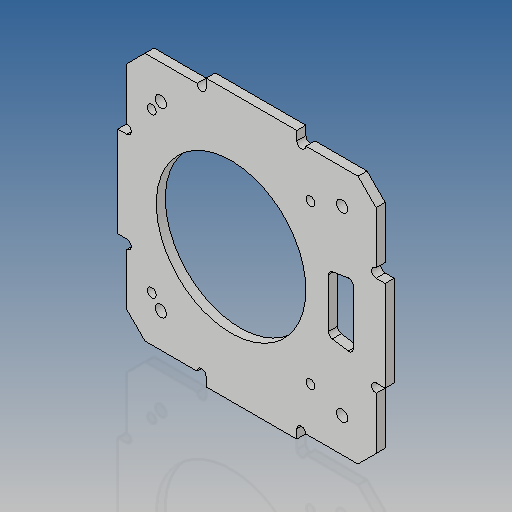
# Autodesk Inventor part: Pieza4
Saved by Autodesk Inventor 2017 (Build 210142000, 142)
## iProperties
Part Number: Pieza4
Material: Genérico
Document SubType Name: Modeling
Designer: Leo
Density: 1 g/cm^3
Appearance: Valor por defecto
Author: Leo
Autodesk Inventor part; units mm, degrees
ref_plane "YZ Plane" through (0, 0, 0) normal (1, 0, 0) x (0, 1, 0)
ref_plane "XZ Plane" through (0, 0, 0) normal (0, 1, 0) x (-1, 0, 0)
ref_plane "XY Plane" through (0, 0, 0) normal (0, 0, 1) x (1, 0, 0)
sketch "Boceto1" plane through (0, 0, 0) normal (0, 0, 1) x (1, 0, 0)
  line L0 (32.5, 7.5) -> (0.5, 7.5) construction
  line L1 (0.5, 7.5) -> (0.5, 31.5) construction
  line L2 (0.5, 31.5) -> (32.5, 31.5) construction
  line L3 (32.5, 31.5) -> (32.5, 7.5) construction
  line L4 (30, -12) -> (30, -31) construction
  line L5 (30, -31) -> (3, -31) construction
  line L6 (3, -31) -> (3, -12) construction
  line L7 (3, -12) -> (30, -12) construction
  circle A0 centre (-40, -40) radius 2.5 projected
  circle A1 centre (-40, 40) radius 2.5 projected
  circle A2 centre (40, 40) radius 2.5 projected
  circle A3 centre (40, -40) radius 2.5 projected
  line L8 (-59, 20) -> (-59, -20) projected
  line L9 (-59, -20) -> (-55, -20) projected
  arc A4 (-55, -24) -> (-55, -20) centre (-55, -22) ccw projected
  line L10 (-55, -24) -> (-55, -47) projected
  line L11 (-55, -47) -> (-47, -55) projected
  line L12 (-47, -55) -> (-24, -55) projected
  arc A5 (-20, -55) -> (-24, -55) centre (-22, -55) ccw projected
  line L13 (-20, -55) -> (-20, -59) projected
  line L14 (-20, -59) -> (20, -59) projected
  line L15 (20, -59) -> (20, -55) projected
  arc A6 (24, -55) -> (20, -55) centre (22, -55) ccw projected
  line L16 (24, -55) -> (47, -55) projected
  line L17 (47, -55) -> (55, -47) projected
  line L18 (55, -47) -> (55, -24) projected
  arc A7 (55, -20) -> (55, -24) centre (55, -22) ccw projected
  line L19 (55, -20) -> (59, -20) projected
  line L20 (59, -20) -> (59, 20) projected
  line L21 (59, 20) -> (55, 20) projected
  arc A8 (55, 24) -> (55, 20) centre (55, 22) ccw projected
  line L22 (55, 24) -> (55, 47) projected
  line L23 (55, 47) -> (47, 55) projected
  line L24 (47, 55) -> (24, 55) projected
  arc A9 (20, 55) -> (24, 55) centre (22, 55) ccw projected
  line L25 (20, 55) -> (20, 59) projected
  line L26 (20, 59) -> (-20, 59) projected
  line L27 (-20, 59) -> (-20, 55) projected
  arc A10 (-24, 55) -> (-20, 55) centre (-22, 55) ccw projected
  line L28 (-24, 55) -> (-47, 55) projected
  line L29 (-47, 55) -> (-55, 47) projected
  line L30 (-55, 47) -> (-55, 24) projected
  arc A11 (-55, 20) -> (-55, 24) centre (-55, 22) ccw projected
  line L31 (-55, 20) -> (-59, 20) projected
  line L32 (26, 35) -> (-44, 35) construction
  line L33 (-44, 35) -> (-44, -35) construction
  line L34 (-44, -35) -> (26, -35) construction
  line L35 (26, -35) -> (26, 35) construction
  circle A12 centre (26, 35) radius 2
  circle A13 centre (26, -35) radius 2
  circle A14 centre (-44, -35) radius 2
  circle A15 centre (-44, 35) radius 2
  circle A16 centre (-9, 0) radius 33
  line L36 (45, 12) -> (45, -12)
  arc A17 (42.6827, -13.9747) -> (45, -12) centre (43, -12) ccw
  line L37 (42.6827, -13.9747) -> (35.6827, -12.85)
  arc A18 (34, -10.8753) -> (35.6827, -12.85) centre (36, -10.8753) ccw
  line L38 (34, -10.8753) -> (34, 10.8753)
  arc A19 (35.6827, 12.85) -> (34, 10.8753) centre (36, 10.8753) ccw
  line L39 (35.6827, 12.85) -> (42.6827, 13.9747)
  arc A20 (45, 12) -> (42.6827, 13.9747) centre (43, 12) ccw
  point P0 (26, 0)
  point P1 (59, 0)
  point P2 (-9, 35)
  point P3 (34, 0)
  point P4 (45, 0)
  dimension "d0" = 70
  dimension "d1" = 4
  dimension "d2" = 66
  dimension "d3" = 2
  dimension "d4" = 11
  dimension "d5" = 28
  dimension "d6" = 25.7
  dimension "d7" = 11
  dimension "d8" = 8
  constraints: 16 end point, 9 centre point, 8 point on circle, 8 tangent, 6 equal radius, 5 midpoint, 4 coincident, 4 horizontal alignment, 3 parallel, 2 perpendicular, 1 horizontal, 1 vertical, 1 vertical alignment
  measures "d0" distance of L32.start L32.end
  measures "d1" diameter of A12
  measures "d2" diameter of A16
  measures "d3" radius of A19
  measures "d4" distance between parallel lines of L36 L38
  measures "d6" distance of L39.start L37.end
  measures "d7" distance between parallel lines of L33 L30
  measures "d8" distance between parallel lines of L38 L35
extrude "Extrusión1" add sketch "Boceto1" along normal blind 4
